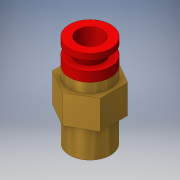
# Autodesk Inventor part: am-2010
Saved by Autodesk Inventor 2016 SP2 (Build 200236200, 236)
## iProperties
Created: 2017-03-28
Part Number: am-2010
Material: Brass
Document SubType Name: Modeling
Designer: smiku
Mass: 15.4259 g
Surface Area: 18.1983 cm^2
Volume: 1.81695 cm^3
Density: 8.49 g/cm^3
Appearance: Brass - Polished
Author: smiku
Autodesk Inventor part; units mm, degrees
ref_plane "YZ Plane" through (0, 0, 0) normal (1, 0, 0) x (0, 1, 0)
ref_plane "XZ Plane" through (0, 0, 0) normal (0, 1, 0) x (-1, 0, 0)
ref_plane "XY Plane" through (0, 0, 0) normal (0, 0, 1) x (1, 0, 0)
sketch "Sketch1" plane through (0, 0, 0) normal (0, 1, 0) x (-1, 0, 0)
  circle A0 centre (0, 0) radius 6.3373 construction
  line L0 (6.3373, -3.6588) -> (0, -7.3177)
  line L1 (0, -7.3177) -> (-6.3373, -3.6588)
  line L2 (-6.3373, -3.6588) -> (-6.3373, 3.6588)
  line L3 (-6.3373, 3.6588) -> (0, 7.3177)
  line L4 (0, 7.3177) -> (6.3373, 3.6588)
  line L5 (6.3373, 3.6588) -> (6.3373, -3.6588)
  circle A1 centre (0, 0) radius 3.2639
  point P0 (6.3373, 0)
  dimension "d0" = 12.6746
  dimension "d1" = 6.5278
  constraints: 12 end point, 3 coincident, 1 centre point, 1 horizontal alignment, 1 midpoint, 1 vertical, 15 other
  measures "d1" diameter of A1
extrude "Extrusion1" add sketch "Sketch1" along normal mid plane 7.62
sketch "Sketch2" plane through (0, 3.81, 0) normal (0, 1, 0) x (1, 0, 0)
  circle A0 centre (0, 0) radius 5.4864
  circle A1 centre (0, 0) radius 3.2639 projected
  dimension "d4" = 10.9728
  constraints: 1 centre point, 1 coincident
  measures "d4" diameter of A0
extrude "Extrusion2" add sketch "Sketch2" along normal blind 2.54
sketch "Sketch3" plane through (0, -3.81, 0) normal (0, -1, 0) x (1, 0, 0)
  circle A0 centre (0, 0) radius 5.4229
  circle A1 centre (0, 0) radius 2.286
  dimension "d7" = 10.8458
  dimension "d8" = 4.572
  constraints: 2 centre point, 2 coincident
  measures "d7" diameter of A0
  measures "d8" diameter of A1
extrude "Extrusion3" add sketch "Sketch3" along normal blind 7.747
sketch "Sketch4" plane through (0, 6.35, 0) normal (0, 1, 0) x (1, 0, 0)
  circle A0 centre (0, 0) radius 3.2639 projected
  circle A1 centre (0, 0) radius 5.4864 projected
extrude "Extrusion4" add sketch "Sketch4" along normal blind 2.54 separate body
sketch "Sketch5" plane through (0, 8.89, 0) normal (0, 1, 0) x (1, 0, 0)
  circle A0 centre (0, 0) radius 3.2639 projected
  circle A1 centre (0, 0) radius 3.5433
  dimension "d13" = 7.0866
  constraints: 1 centre point, 1 coincident
  measures "d13" diameter of A1
extrude "Extrusion5" add sketch "Sketch5" along normal blind 2.54 bodies 2
sketch "Sketch6" plane through (0, 11.43, 0) normal (0, 1, 0) x (1, 0, 0)
  circle A0 centre (0, 0) radius 3.2639 projected
  circle A1 centre (0, 0) radius 5.4864 projected
extrude "Extrusion6" add sketch "Sketch6" along normal blind 1.6002 bodies 2
body "Solid1"
body "Solid2"
